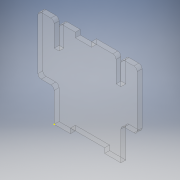
# Autodesk Inventor part: front_left_v2
Saved by Autodesk Inventor 2017.2 (Build 212233000, 233)
## iProperties
Created: 2017-06-09
Part Number: front_left_v2
Material: Generic
Document SubType Name: Modeling
Designer: SandeepSH
Density: 1 g/cm^3
Appearance: Polycarbonate - Clear
Author: SandeepSH
Autodesk Inventor part; units mm, degrees
ref_plane "YZ Plane" through (0, 0, 0) normal (1, 0, 0) x (0, 1, 0)
ref_plane "XZ Plane" through (0, 0, 0) normal (0, 1, 0) x (-1, 0, 0)
ref_plane "XY Plane" through (0, 0, 0) normal (0, 0, 1) x (1, 0, 0)
sketch "Sketch1" plane through (0, 0, 0) normal (0, 0, 1) x (1, 0, 0)
  line L0 (0, 0) -> (41, 0)
  line L1 (41, 0) -> (41, 55.5)
  line L2 (41, 55.5) -> (0, 55.5)
  line L3 (0, 55.5) -> (0, 0)
  dimension "d0" = 41
  dimension "d1" = 55.5
  constraints: 8 end point, 2 parallel, 1 horizontal, 1 perpendicular
  measures "d0" distance of L2.end L1.end
  measures "d1" distance of L1.end L0.end
extrude "Extrusion1" add sketch "Sketch1" along normal blind 3
sketch "Sketch2" plane through (0, 0, 3) normal (0, 0, 1) x (1, 0, 0)
  line L0 (0, 0) -> (41, 0) projected
  line L1 (0, 55.5) -> (0, 0) projected
  line L2 (41, 0) -> (41, 55.5) projected
  line L3 (41, 55.5) -> (0, 55.5) projected
  line L4 (0, 0) -> (10, 0)
  line L5 (10, 0) -> (10, 3)
  line L6 (10, 3) -> (0, 3)
  line L7 (0, 3) -> (0, 0)
  line L8 (41, 0) -> (31, 0)
  line L9 (31, 0) -> (31, 3)
  line L10 (31, 3) -> (41, 3)
  line L11 (41, 3) -> (41, 0)
  line L12 (13, 52.5) -> (23, 52.5)
  line L13 (23, 52.5) -> (23, 55.5)
  line L14 (23, 55.5) -> (13, 55.5)
  line L15 (13, 55.5) -> (13, 52.5)
  line L16 (13, 52.5) -> (23, 55.5) construction
  line L17 (23, 52.5) -> (13, 55.5) construction
  line L18 (13, 52.5) -> (23, 52.5) construction
  line L19 (10, 0) -> (31, 0)
  line L20 (31, 0) -> (31, 3)
  line L21 (31, 3) -> (10, 3)
  line L22 (10, 3) -> (10, 0)
  point P0 (18, 54)
  dimension "d35" = 10
  dimension "d36" = 3
  dimension "d37" = 10
  dimension "d38" = 3
  dimension "d39" = 10
  dimension "d40" = 0
  dimension "d41" = 3
  constraints: 38 end point, 9 parallel, 4 horizontal, 4 perpendicular, 2 collinear, 2 midpoint
  measures "d35" distance of L6.end L5.end
  measures "d36" distance of L5.end L4.end
  measures "d37" distance of L9.end L10.end
  measures "d38" distance of L8.end L9.end
  measures "d39" distance of L12.start L12.end
  measures "d40" distance between parallel lines of L12 L18
  measures "d41" distance of L13.end L12.end
sketch "Sketch3" plane through (0, 0, 3) normal (0, 0, 1) x (1, 0, 0)
  line L0 (41, 0) -> (41, 55.5) projected
  line L1 (41, 55.5) -> (38, 55.5)
  line L2 (38, 55.5) -> (38, 40.5)
  line L3 (38, 40.5) -> (41, 40.5)
  line L4 (41, 40.5) -> (41, 55.5)
  point P0 (0, 0)
  dimension "d16" = 3
  dimension "d17" = 15
  constraints: 8 end point, 2 parallel, 1 horizontal, 1 perpendicular
  measures "d16" distance of L3.end L2.end
  measures "d17" distance of L2.end L1.end
extrude "Extrusion3" cut sketch "Sketch3" against normal through all
sketch "Sketch4" plane through (0, 0, 3) normal (0, 0, 1) x (1, 0, 0)
  line L0 (38, 55.5) -> (0, 55.5) projected
  line L1 (41, 0) -> (41, 40.5) projected
  line L2 (41, 20) -> (51, 20)
  line L3 (51, 20) -> (51, 55.5)
  line L4 (51, 55.5) -> (41, 55.5)
  line L5 (41, 55.5) -> (41, 20)
  line L6 (0, 0) -> (41, 0) projected
  point P0 (69, 46)
  point P1 (89, 0)
  point P2 (0, 55.5)
  dimension "d20" = 10
  dimension "d21" = 20
  constraints: 8 end point, 2 horizontal, 2 parallel, 1 perpendicular, 1 point on line, 1 other
  measures "d20" distance of L4.end L3.end
  measures "d21" distance between parallel lines of L2 L6
extrude "Extrusion4" add sketch "Sketch4" against normal blind 3
sketch "Sketch5" plane through (0, 0, 3) normal (0, 0, 1) x (1, 0, 0)
  line L0 (0, 55.5) -> (0, 0) projected
  line L1 (0, 55.5) -> (-10, 55.5)
  line L2 (-10, 55.5) -> (-10, 20)
  line L3 (-10, 20) -> (0, 20)
  line L4 (0, 20) -> (0, 55.5)
  line L5 (0, 0) -> (41, 0) projected
  point P0 (20, 0)
  dimension "d24" = 10
  dimension "d25" = 20
  constraints: 8 end point, 2 parallel, 1 horizontal, 1 perpendicular
  measures "d24" distance of L3.end L2.end
  measures "d25" distance between parallel lines of L5 L3
extrude "Extrusion5" add sketch "Sketch5" against normal blind 3
sketch "Sketch6" plane through (0, 0, 3) normal (0, 0, 1) x (1, 0, 0)
  point P0 (0, 0)
sketch "Sketch7" plane through (0, 0, 3) normal (0, 0, 1) x (1, 0, 0)
  line L0 (38, 55.5) -> (-10, 55.5) projected
  line L1 (0, 55.5) -> (3, 55.5)
  line L2 (3, 55.5) -> (3, 40.5)
  line L3 (3, 40.5) -> (0, 40.5)
  line L4 (0, 40.5) -> (0, 55.5)
  point P0 (0, 0)
  point P1 (30, 46)
  point P2 (-10, 55.5)
  dimension "d28" = 3
  dimension "d29" = 15
  constraints: 8 end point, 2 parallel, 1 horizontal, 1 perpendicular, 2 other
  measures "d28" distance of L2.end L3.end
  measures "d29" distance of L1.end L2.end
extrude "Extrusion6" cut sketch "Sketch7" against normal through all
fillet "Fillet1" radius 2 10 edges at (0, 55.5, 1.5) (3, 55.5, 1.5) (-10, 55.5, 1.5) (38, 55.5, 1.5) (41, 55.5, 1.5) (51, 55.5, 1.5) (51, 20, 1.5) (41, 20, 1.5) (-10, 20, 1.5) (0, 20, 1.5)
extrude "Extrusion7" cut sketch "Sketch2" against normal through all contours L5 L21 L9 L0 | L3 L13 L12 L15
body "Solid1"
